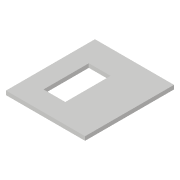
# Autodesk Inventor part: SwitchMount
Saved by Autodesk Inventor 2018 (Build 220112000, 112)
## iProperties
Created: 2017-12-14
Part Number: SwitchMount
Material: Generic
Document SubType Name: Modeling
Designer: ball
Density: 1 g/cm^3
Appearance: Default
Author: ball
Autodesk Inventor part; units mm, degrees
ref_plane "YZ Plane" through (0, 0, 0) normal (1, 0, 0) x (0, 1, 0)
ref_plane "XZ Plane" through (0, 0, 0) normal (0, 1, 0) x (-1, 0, 0)
ref_plane "XY Plane" through (0, 0, 0) normal (0, 0, 1) x (1, 0, 0)
sketch "Sketch1" plane through (0, 0, 0) normal (0, 1, 0) x (-1, 0, 0)
  line L0 (0, 0) -> (-50.8, 0)
  line L1 (-50.8, 0) -> (-50.8, -57.15)
  line L2 (-50.8, -57.15) -> (0, -57.15)
  line L3 (0, -57.15) -> (0, 0)
  dimension "d0" = 50.8
  dimension "d1" = 57.15
  constraints: 8 end point, 2 parallel, 1 horizontal, 1 perpendicular
  measures "d0" distance of L2.end L1.end
  measures "d1" distance of L1.end L0.end
extrude "Extrusion1" add sketch "Sketch1" along normal blind 2.54
sketch "Sketch2" plane through (0, 2.54, 0) normal (0, 1, 0) x (1, 0, 0)
  line L0 (11.43, 12.7) -> (25.4, 12.7)
  line L1 (25.4, 12.7) -> (25.4, 41.783)
  line L2 (25.4, 41.783) -> (11.43, 41.783)
  line L3 (11.43, 41.783) -> (11.43, 12.7)
  line L4 (0, 0) -> (50.8, 0) projected
  point P0 (12.7, 25.4)
  dimension "d4" = 13.97
  dimension "d5" = 29.083
  dimension "d6" = 12.7
  dimension "d7" = 25.4
  constraints: 8 end point, 2 parallel, 1 coincident, 1 horizontal, 1 perpendicular
  measures "d4" distance of L2.end L1.end
  measures "d5" distance of L1.end L0.end
  measures "d6" distance from line of L4 L0.end
  measures "d7" horizontal distance of L4.end L0.end
extrude "Extrusion2" cut sketch "Sketch2" against normal blind 2.54
body "Solid1"
